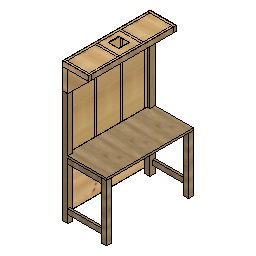
Workbench (Autodesk Fusion 360 design; units mm, degrees)
Autodesk Fusion 360 part; units mm, degrees
box "BoxPrimitive1" add length 774.7 width 469.9 height 469.9 placed x (0, 1, 0) y (-1, 0, 0) z (0, 0, 1) at (469.9, 0, 0) makes body 1
box "BoxPrimitive2" add length 508 width 609.6 height 977.9 placed x (0, -1, 0) y (1, 0, 0) z (0, 0, 1) at (0, 0, 0) separate body makes body 2
sketch "4x4" plane through (0, 0, 0) normal (0, 0, 1) x (1, 0, 0)
  line L0 (0, 0) -> (88.9, 0)
  line L1 (88.9, 0) -> (88.9, -88.9)
  line L2 (88.9, -88.9) -> (0, -88.9)
  line L3 (0, -88.9) -> (0, 0)
  dimension "d22" = 88.9
  dimension "d23" = 88.9
  constraint horizontal L0
  constraint vertical L1
  constraint horizontal L2
  constraint vertical L3
  constraint coincident L0.start L3.end
  measures "d22" distance of L0.start L0.end
  measures "d23" distance of L0.start L2.end
extrude "Extrude1" add sketch "4x4" along normal blind 2336.8 separate body makes body 3 in component "Bench"
move_body "Move1" bodies 1 to x (1, 0, 0) y (0, 1, 0) z (0, 0, 1) at (0, 25.4, 0)
move_body "Move2" bodies 1 to x (1, 0, 0) y (0, 1, 0) z (0, 0, 1) at (0, 393.7, 0)
move_body "Move3" bodies 2 to x (1, 0, 0) y (0, 1, 0) z (0, 0, 1) at (0, 508, 0)
move_body "Move4" bodies 2 to x (1, 0, 0) y (0, 1, 0) z (0, 0, 1) at (0, 25.4, 0)
move_body "Move5" bodies 1 to x (1, 0, 0) y (0, 1, 0) z (0, 0, 1) at (0, 139.7, 0)
copy_body "CopyPasteBodies1" bodies 3 makes body 4 in component "Bench"
move_body "Move1'" bodies 4 to x (1, 0, 0) y (0, 1, 0) z (0, 0, 1) at (0, -1435.1, 0) in component "Bench"
move_body "Move6" bodies 2 to x (1, 0, 0) y (0, 1, 0) z (0, 0, 1) at (0, 76.2, 0)
move_body "Move7" bodies 1 to x (1, 0, 0) y (0, 1, 0) z (0, 0, 1) at (0, 88.9, 0)
move_body "Move8" bodies 1 to x (1, 0, 0) y (0, 1, 0) z (0, 0, 1) at (88.9, 0, 0)
move_body "Move9" bodies 2 to x (1, 0, 0) y (0, 1, 0) z (0, 0, 1) at (88.9, 0, 0)
ref_plane "WorkPlane1" through (0, 0, 990.6) normal (0, 0, 1) x (1, 0, 0) in component "Bench"
box "BoxPrimitive1'" add length 1524 width 762 height 38.1 placed x (0, -1, 0) y (1, 0, 0) z (0, 0, 1) at (0, 0, 990.6) bodies 3 4 in component "Bench"
box "BoxPrimitive2'" add length 88.9 width 88.9 height 990.6 placed x (0, 1, 0) y (-1, 0, 0) z (0, 0, 1) at (765.3244, -1514.7947, 0) separate body makes body 5 in component "Bench"
move_body "Move2'" bodies 5 to x (1, 0, 0) y (0, 1, 0) z (0, 0, 1) at (-3.3244, -9.2053, 0) in component "Bench"
copy_body "CopyPasteBodies2" bodies 5 makes body 6 in component "Bench"
move_body "Move3'" bodies 6 to x (1, 0, 0) y (0, 1, 0) z (0, 0, 1) at (0, 1435.1, 0) in component "Bench"
ref_plane "WorkPlane2" through (0, 0, 2540) normal (0, 0, 1) x (1, 0, 0) in component "Bench"
box "BoxPrimitive3" add length 88.9 width 38.1 height 457.2 placed x (0, 0, 1) y (0, 1, 0) z (-1, 0, 0) at (0, -1524, 2438.4) separate body makes body 7 in component "Bench"
move_body "Move4'" bodies 7 to x (1, 0, 0) y (0, 1, 0) z (0, 0, 1) at (457.2, 0, 0) in component "Bench"
copy_body "CopyPasteBodies3" bodies 7 makes body 8 in component "Bench"
move_body "Move5'" bodies 8 to x (1, 0, 0) y (0, 1, 0) z (0, 0, 1) at (0, 0, 101.6) in component "Bench"
move_body "Move6'" bodies 8 to x (1, 0, 0) y (0, 1, 0) z (0, 0, 1) at (0, 1485.9, -203.2) in component "Bench"
move_body "Move7'" bodies 7 to x (1, 0, 0) y (0, 1, 0) z (0, 0, 1) at (0, 0, -101.6) in component "Bench"
box "BoxPrimitive4" add length 88.9 width 38.1 height 1447.8 placed x (0, 0, -1) y (1, 0, 0) z (0, -1, 0) at (0, -38.1, 2425.7) separate body makes body 9 in component "Bench"
copy_body "CopyPasteBodies4" bodies 9 makes body 10 in component "Bench"
move_body "Move8'" bodies 10 to x (1, 0, 0) y (0, 1, 0) z (0, 0, 1) at (419.1, 0, 0) in component "Bench"
box "BoxPrimitive5" add length 715 width 665 height 720 placed x (0, -1, 0) y (1, 0, 0) z (0, 0, 1) at (146.5643, -88.9, 1028.7) separate body makes body 11 in component "Bench"
copy_body "CutPasteBodies1" bodies 11 body 11 seen with x (1, 0, 0) y (0, 1, 0) z (0, 0, 1) at (0, 1524, 0) removing the originals makes body 12
move_body "Move10" bodies 12 to x (1, 0, 0) y (0, 1, 0) z (0, 0, 1) at (-49.5643, 88.9, 0)
box "BoxPrimitive6" add length 200 width 200 height 410 placed x (0, 1, 0) y (-1, 0, 0) z (0, 0, 1) at (346.84, -1435.1, 1028.7) separate body makes body 13 in component "Bench"
copy_body "CutPasteBodies2" bodies 13 body 13 seen with x (1, 0, 0) y (0, 1, 0) z (0, 0, 1) at (0, 1524, 0) removing the originals makes body 14
box "BoxPrimitive7" add length 200 width 200 height 352 placed x (0, 1, 0) y (-1, 0, 0) z (0, 0, 1) at (400, -1200, 1028.7) separate body makes body 15 in component "Bench"
move_body "Move9'" bodies 15 to x (1, 0, 0) y (0, 1, 0) z (0, 0, 1) at (-50, 0, 0) in component "Bench"
copy_body "CutPasteBodies3" bodies 15 body 15 seen with x (1, 0, 0) y (0, 1, 0) z (0, 0, 1) at (0, 1524, 0) removing the originals makes body 16
box "BoxPrimitive8" add length 88.9 width 38.1 height 381 placed x (0, 0, -1) y (0, 1, 0) z (1, 0, 0) at (38.1, -1029.8346, 2425.7) separate body makes body 17 in component "Bench"
move_body "Move10'" bodies 17 to x (1, 0, 0) y (0, 1, 0) z (0, 0, 1) at (0, 39.2346, 0) in component "Bench"
copy_body "CopyPasteBodies5" bodies 17 makes body 18 in component "Bench"
move_body "Move11" bodies 18 to x (1, 0, 0) y (0, 1, 0) z (0, 0, 1) at (0, 419.1, 0) in component "Bench"
box "BoxPrimitive9" add length 1524 width 457.2 height 5.2 placed x (0, 1, 0) y (-1, 0, 0) z (0, 0, 1) at (457.2, -1524, 2425.7) separate body makes body 19 in component "Bench"
box "BoxPrimitive10" add length 2336.8 width 1524 height 5.2 placed x (0, 0, -1) y (0, -1, 0) z (-1, 0, 0) at (0, 0, 2425.7) separate body makes body 20 in component "Bench"
sketch "CanopySideSketch" plane through (0, -1524, 0) normal (0, -1, 0) x (1, 0, 0) in component "Bench"
  line L0 (0, 2336.8) -> (457.2, 2336.8)
  line L1 (457.2, 2336.8) -> (457.2, 2425.7)
  line L2 (457.2, 2425.7) -> (0, 2425.7)
  line L3 (0, 2425.7) -> (0, 2336.8)
  line L4 (0, 2425.7) -> (457.2, 2425.7)
  line L5 (0, 2425.7) -> (0, 1968.5)
  line L6 (457.2, 2425.7) -> (457.2, 2331.6)
  line L7 (0, 1968.5) -> (88.9, 1968.5)
  line L8 (88.9, 1968.5) -> (457.2, 2331.6)
  dimension "d119" = 457.2
  dimension "d120" = 457.2
  dimension "d121" = 94.1
  dimension "d122" = 88.9
  constraint horizontal L4
  constraint coincident L2.end L3.start
  constraint perpendicular L0 L5
  constraint coincident L1.end L2.start
  constraint perpendicular L0 L6
  constraint perpendicular L5 L7
  measures "d119" distance of L2.end L1.end
  measures "d120" distance of L2.end L5.end
  measures "d121" distance of L1.end L6.end
  measures "d122" distance of L5.end L7.end
extrude "Extrude2" add sketch "CanopySideSketch" along normal blind 5.2 separate body makes body 21 in component "Bench"
move_body "Move12" bodies 21 to x (1, 0, 0) y (0, 1, 0) z (0, 0, 1) at (0, 0, 5.2) in component "Bench"
copy_body "CopyPasteBodies6" bodies 21 makes body 22 in component "Bench"
move_body "Move13" bodies 22 to x (1, 0, 0) y (0, 1, 0) z (0, 0, 1) at (0, 1529.2, 0) in component "Bench"
box "BoxPrimitive11" add length 88.9 width 38.1 height 1346.2 placed x (0, 0, -1) y (1, 0, 0) z (0, -1, 0) at (0, -88.9, 990.6) separate body makes body 23 in component "Bench"
box "BoxPrimitive12" add length 88.9 width 38.1 height 584.2 placed x (0, 0, -1) y (0, 1, 0) z (1, 0, 0) at (88.9, -1524, 990.6) separate body makes body 24 in component "Bench"
copy_body "CopyPasteBodies7" bodies 24 makes body 25 in component "Bench"
move_body "Move14" bodies 25 to x (1, 0, 0) y (0, 1, 0) z (0, 0, 1) at (0, 0, -762) in component "Bench"
copy_body "CopyPasteBodies8" bodies 24 25 makes body 26 makes body 27 in component "Bench"
move_body "Move15" bodies 26 27 to x (1, 0, 0) y (0, 1, 0) z (0, 0, 1) at (0, 1485.9, 0) in component "Bench"
move_body "Move11'" bodies 12 to x (1, 0, 0) y (0, 1, 0) z (0, 0, 1) at (0, -88.9, 0)
box "BoxPrimitive14" cut length 184.15 width 184.15 height -5.2 placed x (0, -1, 0) y (-1, 0, 0) z (0, 0, -1) at (305.3998, -666.7498, 2425.7) bodies 19 in component "Bench"
box "BoxPrimitive15" add length 38.1 width 38.1 height 1308.1 placed x (0, -1, 0) y (1, 0, 0) z (0, 0, 1) at (0, -88.9, 1028.7) separate body makes body 28 in component "Bench"
copy_body "CopyPasteBodies9" bodies 28 makes body 29 in component "Bench"
move_body "Move18" bodies 29 to x (1, 0, 0) y (0, 1, 0) z (0, 0, 1) at (0, -1308.1, 0) in component "Bench"
copy_body "CopyPasteBodies10" bodies 29 makes body 30 in component "Bench"
move_body "Move19" bodies 30 to x (1, 0, 0) y (0, 1, 0) z (0, 0, 1) at (0, 457.2, 0) in component "Bench"
copy_body "CopyPasteBodies11" bodies 28 makes body 31 in component "Bench"
move_body "Move20" bodies 31 to x (1, 0, 0) y (0, 1, 0) z (0, 0, 1) at (0, -431.8, 0) in component "Bench"
move_body "Move21" bodies 30 to x (1, 0, 0) y (0, 1, 0) z (0, 0, 1) at (0, -25.4, 0) in component "Bench"
box "BoxPrimitive16" add length 1308.1 width 1346.2 height 4.7625 placed x (0, 0, -1) y (0, 1, 0) z (1, 0, 0) at (38.1, -1435.1, 2336.8) separate body makes body 32 in component "Bench"
sketch "Sketch22" plane through (42.8625, 0, 0) normal (1, 0, 0) x (0, 1, 0) in component "Bench"
  line L0 (-1435.1, 1028.7) -> (-88.9, 1028.7)
  line L1 (-88.9, 1028.7) -> (-88.9, 2336.8)
  line L2 (-88.9, 2336.8) -> (-1435.1, 2336.8)
  line L3 (-1435.1, 2336.8) -> (-1435.1, 1028.7)
  circle A0 centre (-1410, 2310) radius 1.5875
  dimension "d192" = 3.175
  measures "d192" diameter of A0
hole "Hole1" at (42.8625, -1410, 2310) direction (-1, 0, 0) diameter 3.175 depth 6 tip angle 120 bodies 29 32 in component "Bench"
component "Bench" placed x (1, 0, 0) y (0, 1, 0) z (0, 0, 1) at (0, 1524, 0)
equation "d1 = MalleWidth"
equation "d2 = MalleDepth"
equation "d3 = MalleHeight"
equation "d6 = FrigoWidth"
equation "d7 = FrigoDepth"
equation "d8 = FrigoHeight"
equation "Width = 5 ft"
equation "Depth = 30 in"
equation "CounterThickness = 1.5 in"
equation "FrigoHeight = 38.5 in"
equation "FrigoWidth = 20 in"
equation "FrigoDepth = 24 in"
equation "MalleHeight = 18.5 in"
equation "MalleWidth = 30.5 in"
equation "MalleDepth = 18.5 in"
equation "TableHeight = 39 in"
equation "Height = 8 ft - 4 in"
equation "d24 = Height"
equation "d27 = FrigoWidth + 2 in"
equation "d36 = Width - 4 in"
equation "d44 = TableHeight"
equation "d47 = CounterThickness"
equation "d52 = TableHeight"
equation "d55 = Depth"
equation "d59 = Width"
equation "CeilingHeight = 100 in"
equation "d62 = CeilingHeight"
equation "CanopyDepth = 18 in"
equation "d66 = CanopyDepth"
equation "d69 = CanopyDepth"
equation "d77 = Height"
equation "d80 = Width - 3 in"
equation "d100 = CanopyDepth - 3 in"
equation "d104 = -Width / 2 - CanopyDepth / 2"
equation "d107 = -Width / 2 + CanopyDepth / 2"
equation "d119 = CanopyDepth"
equation "d120 = CanopyDepth"
equation "d121 = 3.5 in + 5.2 mm"
equation "d132 = Width - 7 in"
equation "d137 = Depth - 7 in"
equation "d142 = -Depth"
equation "d144 = Width - 1.5 in"
equation "d167 = Height - TableHeight - CounterThickness"
equation "d171 = -Width + 7 in + 1.5 in"
named bodies: "Malle", "Frigo", "FullHeight4x4_right", "FullHeight4x4", "FullHeight4x4_left", "FrontLeftLeg", "FrontRightLeg", "CanopyLeft", "CanopyRight", "CanopyBack", "CanopyFront", "Anycubic Kobra Max", "Elegoo Mars 2 Pro", "Elegoo Mercury Plus 2", "CanopyIntermediateLeft", "CanopyIntermediateRight", "CanopyTop", "Back", "CanopyLeftSide", "CanopyRightSide", "BackTableSupport", "LeftSideTableSupport", "LeftSideFootStructure", "LeftSideTableSupport (1)", "RightSideTableSupport", "RightSideFootStructure", "PegboardSupportRight", "PegboardSupportLeft", "PegboardSupportLeftCenter", "PegboardSupportRight (1)", "PegboardSupportRightCenter", "PegBoard"
